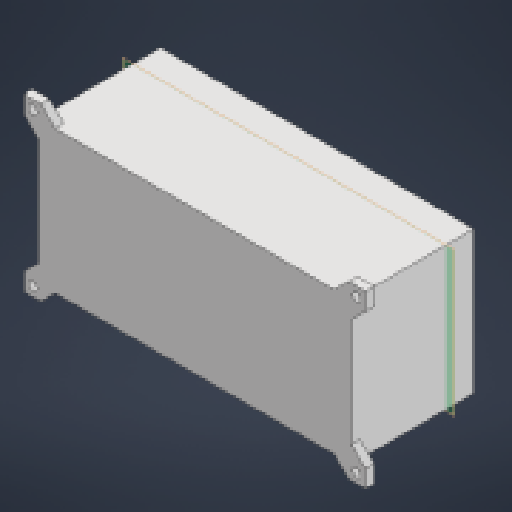
# Autodesk Inventor part: lvl202x01_toggle_body
Saved by Autodesk Inventor 2024 (Build 280153000, 153)
## iProperties
Created: 2026-04-07
Part Number: lvl202x01_toggle_body
Material: Generic
Document SubType Name: Modeling
Designer: schar
Density: 1 g/cm^3
Appearance: Default
Author: schar
Autodesk Inventor part; units mm, degrees
ref_plane "YZ Plane" through (0, 0, 0) normal (1, 0, 0) x (0, 1, 0)
ref_plane "XZ Plane" through (0, 0, 0) normal (0, 1, 0) x (-1, 0, 0)
ref_plane "XY Plane" through (0, 0, 0) normal (0, 0, 1) x (1, 0, 0)
sketch "Sketch1" plane through (0, 0, 0) normal (0, 0, 1) x (1, 0, 0)
  line L0 (-55, 25) -> (55, 25)
  line L1 (55, 25) -> (55, -25)
  line L2 (55, -25) -> (-55, -25)
  line L3 (-55, -25) -> (-55, 25)
  line L4 (-55, 25) -> (55, -25) construction
  line L5 (55, 25) -> (-55, -25) construction
  line L6 (-55, 25) -> (-49, 25)
  line L7 (-60, 30) -> (60, 30)
  line L8 (60, 30) -> (60, -30)
  line L9 (60, -30) -> (-60, -30)
  line L10 (-60, -30) -> (-60, 30)
  line L11 (-60, 30) -> (60, -30) construction
  line L12 (60, 30) -> (-60, -30) construction
  line L13 (-60, 30) -> (-54, 30)
  line L14 (-54, 30) -> (-49, 25)
  line L15 (-55, 25) -> (-55, 19)
  line L16 (-55, 19) -> (-60, 24)
  circle A0 centre (-56.768, 26.768) radius 1.5 projected
  circle A1 centre (-56.768, 26.768) radius 1.5
  line L17 (55, 25) -> (49, 25)
  line L18 (60, 30) -> (54, 30)
  line L19 (54, 30) -> (49, 25)
  line L20 (55, 25) -> (55, 19)
  line L21 (60, 30) -> (60, 24)
  line L22 (60, 24) -> (55, 19)
  line L23 (55, -25) -> (49, -25)
  line L24 (55, -25) -> (55, -19)
  line L25 (60, -30) -> (60, -24)
  line L26 (60, -30) -> (54, -30)
  line L27 (54, -30) -> (49, -25)
  line L28 (55, -19) -> (60, -24)
  line L29 (-55, -25) -> (-49, -25)
  line L30 (-55, -25) -> (-55, -19)
  line L31 (-60, -30) -> (-60, -24)
  line L32 (-60, -24) -> (-55, -19)
  line L33 (-49, -25) -> (-54, -30)
  circle A2 centre (56.768, 26.768) radius 1.5 projected
  circle A3 centre (56.768, -26.768) radius 1.5 projected
  circle A4 centre (-56.768, -26.768) radius 1.5 projected
  point P0 (0, 0)
  dimension "d0" = 110
  dimension "d1" = 50
  dimension "d2" = 6
  dimension "d3" = 120
  dimension "d4" = 60
  dimension "d5" = 6
  dimension "d6" = 6
  dimension "d7" = 6
  dimension "d8" = 6
  dimension "d9" = 6
  dimension "d10" = 6
  dimension "d11" = 6
  dimension "d12" = 6
  dimension "d13" = 6
  dimension "d14" = 6
  dimension "d15" = 6
  dimension "d16" = 6
  constraints: 68 end point, 16 point on line, 6 parallel, 4 midpoint, 2 horizontal, 2 perpendicular, 1 centre point, 1 coincident, 1 concentric
  measures "d0" distance of L1.end L2.end
  measures "d1" distance of L0.end L1.end
  measures "d2" distance of L0.start L6.end
  measures "d3" distance of L8.end L9.end
  measures "d4" distance of L7.end L8.end
  measures "d5" distance of L7.start L13.end
  measures "d6" distance of L0.end L17.end
  measures "d7" distance of L7.end L18.end
  measures "d8" distance of L0.end L20.end
  measures "d9" distance of L7.end L21.end
  measures "d10" distance of L1.end L23.end
  measures "d11" distance of L1.end L24.end
  measures "d12" distance of L8.end L25.end
  measures "d13" distance of L8.end L26.end
  measures "d14" distance of L2.end L29.end
  measures "d15" distance of L2.end L30.end
  measures "d16" distance of L9.end L31.end
extrude "Extrusion1" add sketch "Sketch1" along normal blind 3 contours L3 L16 L10 L7 L14 L0 | L0 L1 L2 L3 | L19 L7 L8 L22 L1 L0 | L3 L2 L33 L9 L10 L32 | L28 L8 L9 L27 L2 L1
sketch "Sketch2" plane through (0, 0, 0) normal (0, 0, -1) x (-1, 0, 0)
  line L0 (-55, 25) -> (55, 25)
  line L1 (55, 25) -> (55, -25)
  line L2 (55, -25) -> (-55, -25)
  line L3 (-55, -25) -> (-55, 25)
  line L4 (-55, 25) -> (55, -25) construction
  line L5 (55, 25) -> (-55, -25) construction
  line L6 (-55, 25) -> (55, 25)
  line L7 (55, 25) -> (55, -25)
  line L8 (55, -25) -> (-55, -25)
  line L9 (-55, -25) -> (-55, 25)
  line L10 (-55, 25) -> (55, -25) construction
  line L11 (55, 25) -> (-55, -25) construction
  line L12 (-53.2, 23.2) -> (53.2, 23.2)
  line L13 (53.2, 23.2) -> (53.2, -23.2)
  line L14 (53.2, -23.2) -> (-53.2, -23.2)
  line L15 (-53.2, -23.2) -> (-53.2, 23.2)
  line L16 (-53.2, 23.2) -> (53.2, -23.2) construction
  line L17 (53.2, 23.2) -> (-53.2, -23.2) construction
  point P0 (0, 0)
  point P1 (-55, -23)
  point P2 (55, -23)
  point P3 (55, 23)
  point P4 (-55, 23)
  point P5 (-53.2, 25)
  point P6 (-53.2, -25)
  point P7 (53.2, -25)
  point P8 (53.2, 25)
  dimension "d19" = 110
  dimension "d20" = 50
  dimension "d21" = 106.4
  dimension "d22" = 46.4
  constraints: 36 end point, 6 midpoint, 6 parallel, 3 horizontal, 3 perpendicular
  measures "d19" distance of L1.end L2.end
  measures "d20" distance of L0.end L1.end
  measures "d21" distance of L13.end L14.end
  measures "d22" distance of L12.end L13.end
extrude "Extrusion2" add sketch "Sketch2" along normal blind 40
ref_plane "Work Plane1" through (0, 0, -30) normal (0, 0, -1) x (-1, 0, 0)
sketch "Sketch7" plane through (0, 0, -30) normal (0, 0, -1) x (-1, 0, 0)
  circle A0 centre (-50.04, 20) radius 1.1 projected
  circle A1 centre (-10.04, 20) radius 1.1 projected
  circle A2 centre (-10.04, -20) radius 1.1 projected
  circle A3 centre (-50.04, -20) radius 1.1 projected
  line L0 (53.2, 23.2) -> (-53.2, 23.2) projected
  line L1 (0, 23.2) -> (0, -23.2)
  line L2 (-53.2, -23.2) -> (53.2, -23.2) projected
  circle A4 centre (50.04, 20) radius 1.1
  circle A5 centre (50.04, -20) radius 1.1
  line L3 (53.2, -23.2) -> (-53.2, -23.2) projected
  line L4 (-46.88, -16.8) -> (-53.2, -16.8)
  line L5 (-53.2, -16.8) -> (-53.2, -23.2)
  line L6 (-53.2, -23.2) -> (-46.88, -23.2)
  line L7 (-46.88, -23.2) -> (-46.88, -16.8)
  line L8 (-46.88, -16.8) -> (-53.2, -23.2) construction
  line L9 (-53.2, -16.8) -> (-46.88, -23.2) construction
  line L10 (-53.2, 23.2) -> (-53.2, -23.2) projected
  line L11 (-46.88, 16.8) -> (-53.2, 16.8)
  line L12 (-53.2, 16.8) -> (-53.2, 23.2)
  line L13 (-53.2, 23.2) -> (-46.88, 23.2)
  line L14 (-46.88, 23.2) -> (-46.88, 16.8)
  line L15 (-46.88, 16.8) -> (-53.2, 23.2) construction
  line L16 (-53.2, 16.8) -> (-46.88, 23.2) construction
  line L17 (-12.7, 16.8) -> (-7.38, 16.8)
  line L18 (-7.38, 16.8) -> (-7.38, 23.2)
  line L19 (-7.38, 23.2) -> (-12.7, 23.2)
  line L20 (-12.7, 23.2) -> (-12.7, 16.8)
  line L21 (-12.7, 16.8) -> (-7.38, 23.2) construction
  line L22 (-7.38, 16.8) -> (-12.7, 23.2) construction
  line L23 (-12.7, -16.8) -> (-7.38, -16.8)
  line L24 (-7.38, -16.8) -> (-7.38, -23.2)
  line L25 (-7.38, -23.2) -> (-12.7, -23.2)
  line L26 (-12.7, -23.2) -> (-12.7, -16.8)
  line L27 (-12.7, -16.8) -> (-7.38, -23.2) construction
  line L28 (-7.38, -16.8) -> (-12.7, -23.2) construction
  line L29 (46.88, 16.8) -> (53.2, 16.8)
  line L30 (53.2, 16.8) -> (53.2, 23.2)
  line L31 (53.2, 23.2) -> (46.88, 23.2)
  line L32 (46.88, 23.2) -> (46.88, 16.8)
  line L33 (46.88, 16.8) -> (53.2, 23.2) construction
  line L34 (53.2, 16.8) -> (46.88, 23.2) construction
  line L35 (46.88, -16.8) -> (53.2, -16.8)
  line L36 (53.2, -16.8) -> (53.2, -23.2)
  line L37 (53.2, -23.2) -> (46.88, -23.2)
  line L38 (46.88, -23.2) -> (46.88, -16.8)
  line L39 (46.88, -16.8) -> (53.2, -23.2) construction
  line L40 (53.2, -16.8) -> (46.88, -23.2) construction
  line L41 (-46.88, 16.8) -> (-46.88, 17.8)
  line L42 (-46.88, 17.8) -> (-53.2, 17.8)
  line L43 (-46.88, 17.8) -> (-47.88, 17.8)
  line L44 (-47.88, 17.8) -> (-47.88, 23.2)
  line L45 (-46.88, -16.8) -> (-47.88, -16.8)
  line L46 (-47.88, -16.8) -> (-47.88, -23.2)
  line L47 (-47.88, -16.8) -> (-47.88, -17.8)
  line L48 (-47.88, -17.8) -> (-53.2, -17.8)
  line L49 (-12.7, -16.8) -> (-12.7, -17.8)
  line L50 (-12.7, -17.8) -> (-7.38, -17.8)
  line L51 (-12.7, 16.8) -> (-12.7, 17.8)
  line L52 (-12.7, 17.8) -> (-7.38, 17.8)
  point P0 (0, 0)
  dimension "d48" = 1
  dimension "d49" = 1
  dimension "d50" = 1
  dimension "d51" = 1
  dimension "d52" = 1
  constraints: 98 end point, 16 point on line, 14 midpoint, 12 parallel, 12 perpendicular, 6 horizontal, 2 centre point, 2 symmetric about line, 2 other
  measures "d48" distance of L11.start L41.end
  measures "d49" distance of L41.end L43.end
  measures "d50" distance of L4.start L45.end
  measures "d51" distance of L45.end L47.end
  measures "d52" distance of L23.start L49.end
extrude "Extrusion6" add sketch "Sketch7" against normal blind 7 contours L30 L29 L32 L0 | L18 L52 L20 L0 | L2 L26 L50 L24 | L44 L42 L10 L0 | L2 L5 L48 L46 | L38 L35 L36 L2
body "Solid1"
